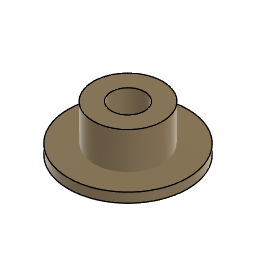
bocaadaptador v4 v1 (Autodesk Fusion 360 design; units mm, degrees)
Autodesk Fusion 360 part; units mm, degrees
sketch "Sketch1" plane through (0, 0, 0) normal (0, 0, 1) x (1, 0, 0)
  circle A0 centre (0, 0) radius 11.99
  dimension "d1" = 23.98
  constraint coincident A0.centre origin
  measures "d1" diameter of A0
sketch "Sketch2" plane through (0, 0, 0) normal (0, 0, 1) x (1, 0, 0)
  circle A0 centre (0, 0) radius 9
  dimension "d2" = 18
  constraint coincident A0.centre origin
  measures "d2" diameter of A0
sketch "Sketch3" plane through (0, 0, 0) normal (0, 1, 0) x (1, 0, 0)
sketch "Sketch4" plane through (0, 0, 0) normal (0, 0, 1) x (1, 0, 0)
  circle A0 centre (0, 0) radius 4.33
  dimension "d3" = 8.66
  constraint coincident A0.centre origin
  measures "d3" diameter of A0
extrude "Extrude1" add sketch "Sketch1" along normal blind 2.49 makes body 1
extrude "Extrude2" add sketch "Sketch2" along normal blind 12 separate body makes body 2
extrude "Extrude3" cut sketch "Sketch4" along normal blind 25 bodies 1 2
sketch "Sketch5" plane through (0, 0, 2.49) normal (0, 0, 1) x (-1, 0, 0)
  circle A0 centre (0, 0) radius 4.33
  circle A1 centre (0, 0) radius 11.99
sketch "Sketch6" plane through (0, 0, 2.49) normal (0, 0, 1) x (-1, 0, 0)
  circle A0 centre (0, 0) radius 15.5
  dimension "d10" = 31
  constraint coincident A0.centre origin
  measures "d10" diameter of A0
extrude "Extrude4" add sketch "Sketch6" against normal blind 2.49 separate body makes body 3
extrude "Extrude5" add sketch "Sketch4" along normal blind 30 separate body makes body 4
sketch "Boceto7" plane through (0, 0, 12) normal (0, 0, 1) x (-1, 0, 0)
  circle A0 centre (0, 0) radius 4.33
  circle A1 centre (0, 0) radius 9
  circle A2 centre (0, 0) radius 4.33
  dimension "d15" = 8.66
  constraint coincident A0.centre A1.centre
  measures "d15" diameter of A2
extrude "Extruir6" cut sketch "Boceto7" against normal blind 13 contours A0 A2 bodies 3
hidden bodies 1 4
named bodies: "Base Botella", "Base alcohol"
